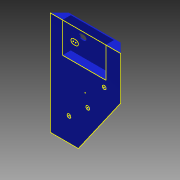
# Autodesk Inventor part: C34_TK_UnderCarriageGuardPlate
Saved by Autodesk Inventor 2015 SP1 (Build 190203100, 203)
## iProperties
Created: 2016-02-10
Part Number: C34_TK_UnderCarriageGuardPlate
Material: Polycarbonate, Clear
Document SubType Name: Modeling
Designer: TheeTimatahee
Density: 1.2 g/cm^3
Appearance: Blue - Wall Paint - Glossy
Author: TheeTimatahee
Autodesk Inventor part; units mm, degrees
ref_plane "YZ Plane" through (0, 0, 0) normal (1, 0, 0) x (0, 1, 0)
ref_plane "XZ Plane" through (0, 0, 0) normal (0, 1, 0) x (-1, 0, 0)
sketch "Sketch1" plane through (0, 0, 0) normal (0, 0, 1) x (1, 0, 0)
  line L0 (-47.625, -69.85) -> (47.625, -69.85)
  line L1 (47.625, -69.85) -> (47.625, 69.85)
  line L2 (47.625, 69.85) -> (-47.625, 69.85)
  line L3 (-47.625, 69.85) -> (-47.625, -69.85)
  line L4 (-47.625, -69.85) -> (47.625, 69.85) construction
  line L5 (47.625, -69.85) -> (-47.625, 69.85) construction
  point P0 (0, 0)
  dimension "d2" = 95.25
  dimension "d3" = 139.7
  constraints: 12 end point, 2 midpoint, 2 parallel, 1 horizontal, 1 perpendicular
  measures "d2" distance of L0.start L0.end
  measures "d3" distance of L2.end L0.start
extrude "Extrusion1" add sketch "Sketch1" along normal blind 12.7
sketch "Sketch5" plane through (0, 0, 0) normal (0, 0, -1) x (-1, 0, 0)
  circle A0 centre (68.072, -112.9665) radius 2.5527 projected
  circle A1 centre (17.272, -112.9665) radius 2.5527 projected
  circle A2 centre (-33.528, -112.9665) radius 2.5527 projected
  circle A3 centre (-84.328, -112.9665) radius 2.5527 projected
  circle A4 centre (-135.128, -112.9665) radius 2.5527 projected
  circle A5 centre (-185.928, -112.9665) radius 2.5527 projected
  circle A6 centre (-211.328, -112.9665) radius 2.5527 projected
  circle A7 centre (-160.528, -112.9665) radius 2.5527 projected
  circle A8 centre (-109.728, -112.9665) radius 2.5527 projected
  circle A9 centre (-58.928, -112.9665) radius 2.5527 projected
  circle A10 centre (-8.128, -112.9665) radius 2.5527 projected
  circle A11 centre (42.672, -112.9665) radius 2.5527 projected
  circle A12 centre (93.472, -112.9665) radius 2.5527 projected
  circle A13 centre (-62.484, -38.6715) radius 3.429 projected
  circle A14 centre (-62.484, 33.7185) radius 3.429 projected
  arc A15 (-54.102, -15.1765) -> (-44.45, -15.1765) centre (-49.276, -15.1765) ccw projected
  line L0 (-44.45, -15.1765) -> (-44.45, 10.2235) projected
  arc A16 (-44.45, 10.2235) -> (-54.102, 10.2235) centre (-49.276, 10.2235) ccw projected
  line L1 (-54.102, 10.2235) -> (-54.102, -15.1765) projected
  arc A17 (-228.854, -15.1765) -> (-219.202, -15.1765) centre (-224.028, -15.1765) ccw projected
  line L2 (-219.202, -15.1765) -> (-219.202, 10.2235) projected
  arc A18 (-219.202, 10.2235) -> (-228.854, 10.2235) centre (-224.028, 10.2235) ccw projected
  line L3 (-228.854, 10.2235) -> (-228.854, -15.1765) projected
  circle A19 centre (-218.3546, -258.6355) radius 2.413 projected
  circle A20 centre (-78.4098, -256.2225) radius 2.413 projected
  circle A21 centre (-78.4098, -297.1165) radius 2.413 projected
  circle A22 centre (-218.3546, -294.7035) radius 2.413 projected
  circle A23 centre (112.522, -87.5665) radius 2.0701 projected
  circle A24 centre (112.522, -138.3665) radius 2.0701 projected
  circle A25 centre (-243.078, 64.8335) radius 2.0701 projected
  circle A26 centre (-243.078, 14.0335) radius 2.0701 projected
  circle A27 centre (-243.078, -36.7665) radius 2.0701 projected
  circle A28 centre (-243.078, -87.5665) radius 2.0701 projected
  circle A29 centre (-243.078, -138.3665) radius 2.0701 projected
  circle A30 centre (-243.078, -189.1665) radius 2.0701 projected
  circle A31 centre (-243.078, -239.9665) radius 2.0701 projected
  circle A32 centre (-243.078, -290.7665) radius 2.0701 projected
  circle A33 centre (-243.078, -265.3665) radius 2.0701 projected
  circle A34 centre (-243.078, -214.5665) radius 2.0701 projected
  circle A35 centre (-243.078, -163.7665) radius 2.0701 projected
  circle A36 centre (-243.078, -112.9665) radius 2.0701 projected
  circle A37 centre (-243.078, -62.1665) radius 2.0701 projected
  circle A38 centre (-243.078, -11.3665) radius 2.0701 projected
  circle A39 centre (-243.078, 39.4335) radius 2.0701 projected
  circle A40 centre (112.522, -163.7665) radius 2.0701 projected
  circle A41 centre (112.522, -112.9665) radius 2.0701 projected
  circle A42 centre (112.522, -62.1665) radius 2.0701 projected
  arc A43 (-45.1979, 77.5335) -> (-51.5479, 83.8835) centre (-51.5479, 77.5335) ccw projected
  line L4 (-45.1979, 77.5335) -> (-45.1979, 54.7638) projected
  arc A44 (-45.1979, 54.7638) -> (-43.3381, 50.2736) centre (-38.8479, 54.7638) ccw projected
  line L5 (-43.3381, 50.2736) -> (29.1422, -22.2066) projected
  arc A45 (31.0021, -26.6968) -> (29.1422, -22.2066) centre (24.6521, -26.6968) ccw projected
  line L6 (31.0021, -26.6968) -> (31.0021, -43.1165) projected
  arc A46 (31.0021, -43.1165) -> (37.3521, -49.4665) centre (37.3521, -43.1165) ccw projected
  line L7 (37.3521, -49.4665) -> (118.872, -49.4665) projected
  line L8 (118.872, -176.4665) -> (118.872, -49.4665) projected
  line L9 (118.872, -176.4665) -> (37.3521, -176.4665) projected
  arc A47 (37.3521, -176.4665) -> (31.0021, -182.8165) centre (37.3521, -182.8165) ccw projected
  line L10 (31.0021, -182.8165) -> (31.0021, -199.2362) projected
  arc A48 (29.1422, -203.7264) -> (31.0021, -199.2362) centre (24.6521, -199.2362) ccw projected
  line L11 (29.1422, -203.7264) -> (-43.3381, -276.2066) projected
  arc A49 (-43.3381, -276.2066) -> (-45.1979, -280.6968) centre (-38.8479, -280.6968) ccw projected
  line L12 (-45.1979, -280.6968) -> (-45.1979, -303.4665) projected
  arc A50 (-51.5479, -309.8165) -> (-45.1979, -303.4665) centre (-51.5479, -303.4665) ccw projected
  line L13 (-249.428, -309.8165) -> (-51.5479, -309.8165) projected
  line L14 (-249.428, 83.8835) -> (-249.428, -309.8165) projected
  line L15 (-51.5479, 83.8835) -> (-249.428, 83.8835) projected
  line L16 (-47.625, -69.85) -> (-47.625, 69.85) projected
  line L17 (47.625, 69.85) -> (47.625, -69.85) projected
  line L18 (47.625, -69.85) -> (-47.625, -69.85) projected
  line L19 (28.575, 28.5877) -> (-28.575, 28.5877) projected
  circle A51 centre (19.05, -44.45) radius 3.3782 projected
  circle A52 centre (-22.225, 19.0627) radius 3.3782 projected
  point P0 (0, 0)
  point P1 (22.225, -38.1)
  point P2 (-25.4, 19.0627)
  point P3 (20.684, -69.85)
  point P4 (-44.45, 19.0627)
  point P5 (19.05, -69.85)
  point P6 (-3.175, -15.875)
  dimension "d47" = 25.4
  dimension "d53" = 22.225
  dimension "d64" = 19.0627
  dimension "d65" = 38.1
  dimension "d108" = 25.4
  dimension "d109" = 53.975
  constraints: 1 other
  measures "d47" distance from line of L17 point (22.225, -38.1)
  measures "d64" vertical distance of point (-25.4, 19.063) point (0, 0)
  measures "d65" vertical distance of point (0, 0) point (22.225, -38.1)
  measures "d108" horizontal distance of point (22.225, -38.1) point (-3.175, -15.875)
  measures "d109" distance from line of L18 point (-3.175, -15.875)
hole "Hole1" at (-22.225, -38.1, 0) at (25.4, 19.0627, 0) at (3.175, -15.875, 0) direction (0, 0, 1) diameter 5.1054 end through all clearance for "Flat Head Machine Screw (82)" size "#10" standard "Ansi Unified Screw Threads"
ref_plane "Work Plane1" through (-41.275, 69.85, 0) normal (0, -1, 0) x (0, 0, -1)
sketch "Sketch7" plane through (0, 0, 12.7) normal (0, 0, 1) x (1, 0, 0)
  line L0 (-9.525, -69.85) -> (47.625, 11.7687)
  line L1 (-47.625, -69.85) -> (47.625, -69.85) projected
  line L2 (-47.625, 69.85) -> (-47.625, -69.85)
  line L3 (47.625, -69.85) -> (47.625, 69.85) projected
  line L4 (47.625, 69.85) -> (-47.625, 69.85) projected
  line L5 (27.625, 69.85) -> (-30.7357, 69.85)
  line L6 (-30.7357, 69.85) -> (-30.7357, 28.5877)
  line L7 (-30.7357, 28.5877) -> (27.625, 28.5877)
  line L8 (-16.7842, 38.1127) -> (14.9658, 38.1127) projected
  line L9 (-16.7842, 50.8127) -> (14.9658, 50.8127) projected
  line L10 (14.9658, 50.8127) -> (14.9658, 38.1127)
  line L11 (-16.7842, 50.8127) -> (-16.7842, 38.1127)
  line L12 (20.4436, 50.8127) -> (24.45, 50.8127) projected
  line L13 (24.0601, 50.8127) -> (24.45, 50.8127) projected
  line L14 (24.0601, 50.8127) -> (-14.952, 50.8127) projected
  line L15 (20.4436, 50.8127) -> (17.9874, 50.8127) projected
  line L16 (-2.2262, 50.8127) -> (17.9874, 50.8127) projected
  line L17 (-2.2262, 52.3875) -> (17.9874, 52.3875) projected
  line L18 (17.9874, 52.3875) -> (20.4436, 52.3875) projected
  line L19 (20.4436, 52.3875) -> (24.45, 52.3875) projected
  line L20 (24.45, 50.8127) -> (24.45, 52.3875) projected
  line L21 (-21.2107, 52.3875) -> (-9.8426, 52.3875) projected
  line L22 (-9.8426, 52.3875) -> (-7.673, 52.3875) projected
  line L23 (-7.673, 52.3875) -> (-5.0722, 52.3875) projected
  line L24 (-5.0722, 52.3875) -> (-2.2262, 52.3875) projected
  line L25 (27.625, 28.5877) -> (27.625, 69.85)
  dimension "d72" = 9.525
  dimension "d73" = 3.175
  dimension "d74" = 9.525
  dimension "d80" = 38.1
  dimension "d84" = 55
  constraints: 16 end point, 3 point on line, 2 perpendicular, 2 vertical, 1 horizontal, 1 parallel
  measures "d72" distance between parallel lines of L8 L7
  measures "d73" distance between parallel lines of L25 L20
  measures "d74" distance from line of L21.start L6
  measures "d80" distance from line of L2 L0.start
  measures "d84" angle of L1 L0
extrude "Extrusion7" cut sketch "Sketch7" against normal blind 11.1125 contours L25 L7 L6 L4 | L11 L9 L10 L8
extrude "Extrusion9" cut sketch "Sketch7" against normal through all contours L0 L3 L1
chamfer "Chamfer3" distance 12.7 angle 45 4 edges at (47.625, 40.8093, 0) (19.05, -29.0407, 0) (-47.625, 0, 0) (-28.575, -69.85, 0)
sketch "Sketch8" plane through (0, 0, 0) normal (0, 0, -1) x (-1, 0, 0)
  line L0 (16.1925, 52.07) -> (13.0175, 52.07) construction
  line L1 (16.1925, 55.4482) -> (13.0175, 55.4482)
  line L2 (13.0175, 48.6918) -> (16.1925, 48.6918)
  arc A0 (16.1925, 48.6918) -> (16.1925, 55.4482) centre (16.1925, 52.07) ccw
  arc A1 (13.0175, 55.4482) -> (13.0175, 48.6918) centre (13.0175, 52.07) ccw
  line L3 (34.925, 69.85) -> (34.925, -57.15) projected
  line L4 (-34.925, 69.85) -> (34.925, 69.85) projected
  point P0 (0, 0)
  point P1 (14.605, 52.07)
  dimension "d88" = 3.3782
  dimension "d89" = 3.175
  dimension "d90" = 20.32
  dimension "d91" = 17.78
  constraints: 8 end point, 4 point on circle, 4 tangent, 2 centre point, 1 horizontal, 1 midpoint, 1 parallel
  measures "d88" radius of A0
  measures "d89" distance of L0.start L0.end
  measures "d90" distance from line of L3 point (14.605, 52.07)
  measures "d91" distance from line of L4 point (14.605, 52.07)
extrude "Extrusion10" cut sketch "Sketch8" against normal blind 11.1125
sketch "Sketch10" plane through (0, 0, 12.7) normal (0, 0, 1) x (1, 0, 0)
  line L0 (-9.525, -69.85) -> (47.625, 11.7687) projected
  line L1 (47.625, 11.7687) -> (47.625, 69.85) projected
  line L2 (47.625, 69.85) -> (27.625, 69.85) projected
  line L3 (27.625, 69.85) -> (27.625, 28.5877) projected
  line L4 (27.625, 28.5877) -> (-30.7357, 28.5877) projected
  line L5 (-30.7357, 28.5877) -> (-30.7357, 69.85) projected
  line L6 (-30.7357, 69.85) -> (-47.625, 69.85) projected
  line L7 (-47.625, 69.85) -> (-47.625, -69.85) projected
  line L8 (-47.625, -69.85) -> (-9.525, -69.85) projected
  circle A0 centre (25.4, 19.0627) radius 2.5527 projected
  circle A1 centre (-22.225, -38.1) radius 2.5527 projected
  circle A2 centre (3.175, -15.875) radius 2.5527 projected
  arc A3 (-13.0175, 48.6918) -> (-13.0175, 55.4482) centre (-13.0175, 52.07) ccw projected
  line L9 (-13.0175, 48.6918) -> (-16.1925, 48.6918) projected
  arc A4 (-16.1925, 55.4482) -> (-16.1925, 48.6918) centre (-16.1925, 52.07) ccw projected
  line L10 (-16.1925, 55.4482) -> (-13.0175, 55.4482) projected
  line L11 (-30.7357, 69.85) -> (27.625, 69.85) projected
  line L12 (-30.7357, 28.5877) -> (-30.7357, 69.85) projected
  line L13 (27.625, 28.5877) -> (-30.7357, 28.5877) projected
  line L14 (27.625, 69.85) -> (27.625, 28.5877) projected
  point P0 (0, 0)
body "Solid1"
